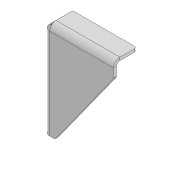
# Autodesk Inventor part: CCM_Mount_C
Saved by Autodesk Inventor 2020 (Build 240168000, 168)
## iProperties
Created: 2021-12-05
Part Number: CCM_Mount_C
Material: 一般
Document SubType Name: Sheet Metal
Designer: ken113
Density: 1 g/cm^3
Sheet Metal Rule: Default_mm
Appearance: 既定
Author: ken113
Autodesk Inventor part; units mm, degrees
ref_plane "YZ Plane" through (0, 0, 0) normal (1, 0, 0) x (0, 1, 0)
ref_plane "XZ Plane" through (0, 0, 0) normal (0, 1, 0) x (-1, 0, 0)
ref_plane "XY Plane" through (0, 0, 0) normal (0, 0, 1) x (1, 0, 0)
sketch "スケッチ1" plane through (0, 0, 0) normal (0, 0, 1) x (1, 0, 0)
  line L0 (30.5, -43.5) -> (-30.5, -43.5)
  line L1 (-30.5, -43.5) -> (-30.5, 43.5)
  line L2 (-30.5, 43.5) -> (30.5, 43.5)
  line L3 (30.5, 43.5) -> (30.5, -43.5)
  line L4 (30.5, -43.5) -> (-30.5, 43.5) construction
  line L5 (-30.5, -43.5) -> (30.5, 43.5) construction
  point P0 (0, 0)
  dimension "d0" = 87
  dimension "d1" = 61
  measures "d0" distance of L0.end L1.end
  measures "d1" distance of L1.end L2.end
extrude "プレート1" add sketch "スケッチ1" along normal blind 3
sketch "スケッチ2" plane through (-33.5, 43.5, -3) normal (-1, 0, 0) x (0, -1, 0)
  line L0 (87, 0) -> (0, 0)
  line L1 (0, 0) -> (0, -16)
  line L2 (0, -16) -> (87, -16)
  line L3 (87, -16) -> (87, 0)
  constraints: 6 end point, 1 horizontal, 1 perpendicular, 1 vertical
edge flange "フランジ1" height 22 angle 90 thickness 3 bend radius 3 thickness toward (-1, 0, 0) relief straight relief width 3 relief depth 1.5 edges at (-30.5, 0, 0) wall of the first edge with corners at (-33.5, -43.5, -3) (-33.5, 43.5, -3) (-33.5, 43.5, -19) (-33.5, -43.5, -19)
bend "曲げ1"
corner "コーナー1"
sketch "スケッチ3" plane through (30.5, 46.5, -3) normal (0, 1, 0) x (-1, 0, 0)
  line L0 (61, 0) -> (0, 0)
  line L1 (0, 0) -> (0, -16)
  line L2 (0, -16) -> (61, -16)
  line L3 (61, -16) -> (61, 0)
  constraints: 6 end point, 1 horizontal, 1 perpendicular, 1 vertical
edge flange "フランジ2" height 22 angle 90 thickness 3 bend radius 3 thickness toward (0, 1, 0) relief straight relief width 3 relief depth 1.5 edges at (0, 43.5, 0) wall of the first edge with corners at (-30.5, 46.5, -3) (30.5, 46.5, -3) (30.5, 46.5, -19) (-30.5, 46.5, -19)
bend "曲げ2"
corner "コーナー2"
sketch "スケッチ4" plane through (0, 0, 3) normal (0, 0, 1) x (1, 0, 0)
  line L0 (30.5, -43.5) -> (-30.5, -43.5) projected
  line L1 (-25.5, -43.5) -> (33.3099, 38.5)
  line L2 (-30.5, -43.5) -> (-30.5, 43.5) projected
  line L3 (-30.5, 43.5) -> (30.5, 43.5) projected
  line L4 (-30.5, -43.5) -> (-30.5, 43.5) projected
  line L5 (30.5, -43.5) -> (-30.5, -43.5) projected
  line L6 (30.5, 43.5) -> (30.5, -43.5) projected
  line L7 (-30.5, 43.5) -> (30.5, 43.5) projected
  point P0 (0, 0)
  point P1 (30.5, 34.5821)
  dimension "d23" = 5
  dimension "d24" = 5
  constraints: 2 end point, 1 point on line
  measures "d23" distance from line of L1.start L2
  measures "d24" distance from line of L3 L1.end
extrude "押し出し1" cut sketch "スケッチ4" against normal through all contours L0 L1 L6
fillet "フィレット1" radius 2 6 edges at (-25.5, -43.5, 1.5) (-35, -43.5, -19) (30.5, 34.5821, 1.5) (30.5, 48, -19) (-35, 43.5, -19) (-30.5, 48, -19)
equation "\"d2\" = Thickness"
equation "\"d3\" = BendReliefWidth"
equation "\"d4\" = BendReliefDepth"
equation "\"d5\" = MinimumRemnant"
equation "\"d6\" = TransitionRadius"
equation "\"d9\" = BendRadius"
equation "\"d10\" = CornerReliefSize"
equation "\"d11\" = GapSize"
equation "\"d12\" = JacobiRadiusSize"
equation "\"d13\" = BendReliefWidth"
equation "\"d14\" = BendReliefDepth"
equation "\"d15\" = MinimumRemnant"
equation "\"d16\" = TransitionRadius"
equation "\"d19\" = BendRadius"
equation "\"d20\" = CornerReliefSize"
equation "\"d21\" = GapSize"
equation "\"d22\" = JacobiRadiusSize"
equation "\"BendRadius\" = Thickness"
equation "\"BendReliefWidth\" = Thickness"
equation "\"BendReliefDepth\" = 0.5 * Thickness"
equation "\"CornerReliefSize\" = 4 * Thickness"
equation "\"MinimumRemnant\" = 2 * Thickness"
equation "\"TransitionRadius\" = BendRadius"
equation "\"JacobiRadiusSize\" = BendRadius"
equation "\"GapSize\" = Thickness"
equation "\"Thickness\" = 3"
